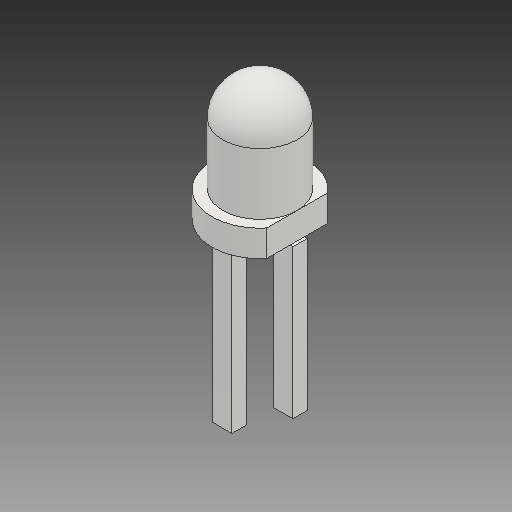
# Autodesk Inventor part: LED 3mm
Saved by Autodesk Inventor 2019.1 (Build 231200000, 200)
## iProperties
Part Number: LED 3mm
Material: PC/ABS-Kunststoff
Document SubType Name: Modeling
Designer: rYan
Density: 0.357273 g/cm^3
Appearance: Glatt - Weiß
Mass: 0.016731 g
Surface Area: 1.09458 cm^2
Volume: 0.0468299 cm^3
Author: rYan
Autodesk Inventor part; units mm, degrees
ref_plane "XZ Plane" through (0, 0, 0) normal (0, 1, 0) x (-1, 0, 0)
ref_plane "XY Plane" through (0, 0, 0) normal (0, 0, 1) x (1, 0, 0)
sketch "Skizze2" plane through (0, 0, 0) normal (0, 1, 0) x (-1, 0, 0)
  line L0 (0, 0) -> (0, 5.2)
  arc A0 (0, 5.2) -> (-1.55, 3.65) centre (0, 3.65) ccw
  line L1 (-1.55, 3.65) -> (-1.55, 1.1)
  line L2 (-1.55, 1.1) -> (-2, 1.1)
  line L3 (-2, 1.1) -> (-2, 0)
  line L4 (-2, 0) -> (0, 0)
  dimension "d0" = 5.2
  dimension "d1" = 3.1
  dimension "d2" = 4.1
  dimension "d3" = 4
  constraints: 10 end point, 3 perpendicular, 2 point on circle, 2 vertical, 1 centre point, 1 point on line, 1 tangent
  measures "d0" distance of L0.start L0.end
  measures "d1" diameter of L1 L0
  measures "d2" distance from line of L2 L0.end
  measures "d3" diameter of L3 L0
revolve "Umdrehung1" add sketch "Skizze2" angle 360 about axis through (0, 0, 0) along (0, 0, 1)
ref_plane "Arbeitsebene1" through (1.55, 0, 2.375) normal (1, 0, 0) x (0, 1, 0)
sketch "Skizze3" plane through (1.55, 0, 2.375) normal (1, 0, 0) x (0, 1, 0)
  line L0 (2, -2.375) -> (-2, -2.375) projected
  line L1 (2, -1.275) -> (-2, -1.275) projected
  line L2 (2, -1.275) -> (-2, -1.275) projected
  line L3 (-2, -1.275) -> (2, -1.275)
  line L4 (2, -1.275) -> (2, -2.375)
  line L5 (2, -2.375) -> (-2, -2.375)
  line L6 (-2, -2.375) -> (-2, -1.275)
  point P0 (0, -2.375)
  constraints: 8 end point, 2 parallel, 1 horizontal, 1 perpendicular
extrude "Extrusion1" cut sketch "Skizze3" along normal through all
sketch "Skizze4" plane through (0, 0, 0) normal (0, 1, 0) x (-1, 0, 0)
  line L0 (-1.55, 0) -> (-1.55, 0) projected
  line L1 (2, 0) -> (-1.55, 0) projected
  line L2 (0.87, 0) -> (1.67, 0)
  line L3 (1.67, 0) -> (1.67, -8)
  line L4 (1.67, -8) -> (0.87, -8)
  line L5 (0.87, -8) -> (0.87, 0)
  line L6 (-1.67, 0) -> (-0.87, 0)
  line L7 (-0.87, 0) -> (-0.87, -6.2)
  line L8 (-0.87, -6.2) -> (-1.67, -6.2)
  line L9 (-1.67, -6.2) -> (-1.67, 0)
  line L10 (0, -7.8775) -> (0, 7.3796) projected
  line L11 (1.27, -8) -> (1.27, 0) construction
  line L12 (-1.27, 0) -> (-1.27, -6.2) construction
  point P0 (0, 0)
  dimension "d7" = 0.8
  dimension "d8" = 0.8
  dimension "d9" = 2.54
  dimension "d10" = 1.8
  dimension "d11" = 8
  constraints: 20 end point, 4 midpoint, 4 parallel, 2 horizontal, 2 perpendicular, 2 point on line, 1 other
  measures "d7" distance of L3.end L4.end
  measures "d8" distance of L7.end L8.end
  measures "d9" distance between parallel lines of L11 L12
  measures "d10" distance between parallel lines of L8 L4
  measures "d11" distance of L2.end L3.end
extrude "Extrusion2" add sketch "Skizze4" along normal mid plane 0.6
sketch "Skizze5" plane through (0, 0, 0) normal (1, 0, 0) x (0, 1, 0)
  line L0 (0, 12.04) -> (0, -35.84) projected
  line L1 (0, 2.4) -> (0, 52.4)
  line L2 (0, 2.4) -> (18.1985, 52.4)
  line L3 (18.1985, 52.4) -> (0, 52.4)
  arc A0 (1.55, 3.65) -> (-1.55, 3.65) centre (0, 3.65) ccw projected
  line L4 (-3.0679, 5.2) -> (3.702, 5.2) construction
  point P0 (0, 0)
  dimension "d14" = 50
  dimension "d15" = 2.8
  dimension "d16" = 20
  constraints: 8 end point, 2 point on line, 1 horizontal, 1 perpendicular, 1 tangent
  measures "d14" distance of L1.start L1.end
  measures "d15" distance from line of L1.start L4
  measures "d16" angle of L2 L1
revolve "Umdrehung2" [suppressed]
